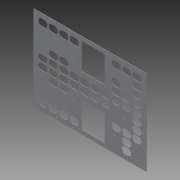
# Autodesk Inventor part: hybridbasearchive
Saved by Autodesk Inventor 2014 SP1 (Build 180222100, 222)
## iProperties
Created: 2014-01-05
Part Number: hybridbasearchive
Material: Aluminum 6061
Document SubType Name: Sheet Metal
Designer: Arpan
Density: 2.71 g/cm^3
Sheet Metal Rule: Default
Appearance: Aluminum - Flat
Mass: 1326.97 g
Surface Area: 6245.09 cm^2
Volume: 489.657 cm^3
Author: Arpan
Autodesk Inventor part; units mm, degrees
(part 1 of 2)
ref_plane "YZ Plane" through (0, 0, 0) normal (1, 0, 0) x (0, 1, 0)
ref_plane "XZ Plane" through (0, 0, 0) normal (0, 1, 0) x (-1, 0, 0)
ref_plane "XY Plane" through (0, 0, 0) normal (0, 0, 1) x (1, 0, 0)
sketch "Sketch1" plane through (0, 0, 0) normal (0, 0, 1) x (1, 0, 0)
  line L0 (0, 0) -> (-685.8, 0)
  line L1 (-685.8, 0) -> (-685.8, 516.255)
  line L2 (-685.8, 516.255) -> (0, 516.255)
  line L3 (0, 516.255) -> (0, 0)
  dimension "d0" = 685.8
  dimension "d1" = 516.255
  measures "d0" distance of L1.end L2.end
  measures "d1" distance of L2.end L0.start
extrude "Plate1" add sketch "Sketch1" along normal blind 1.5875
sketch "Sketch4" plane through (0, 0, 1.5875) normal (0, 0, 1) x (1, 0, 0)
  circle A0 centre (-673.1, 503.555) radius 2.0828 projected
  circle A1 centre (-673.1, 12.7) radius 2.0828 projected
extrude "Cut3" cut sketch "Sketch4" against normal blind 1.5875
pattern_linear "Rectangular Pattern2" count 27 spacing 25.4 along (1, 0, 0) of "Cut3"
sketch "Sketch2" plane through (0, 0, 1.5875) normal (0, 0, 1) x (1, 0, 0)
  line L0 (0, 0) -> (-685.8, 0) projected
  line L1 (-685.8, 516.255) -> (0, 516.255) projected
  line L2 (-342.9, 516.255) -> (-392.43, 516.255)
  line L3 (-392.43, 516.255) -> (-392.43, 332.105)
  line L4 (-392.43, 332.105) -> (-252.73, 332.105)
  line L5 (-252.73, 332.105) -> (-252.73, 516.255)
  line L6 (-392.43, 0) -> (-392.43, 184.15)
  line L7 (-392.43, 184.15) -> (-252.73, 184.15)
  line L8 (-252.73, 184.15) -> (-252.73, 0)
  line L9 (-392.43, 0) -> (-392.43, 25.4)
  line L10 (-392.43, 25.4) -> (-252.73, 25.4)
  line L11 (-252.73, 516.255) -> (-252.73, 490.855)
  line L12 (-252.73, 490.855) -> (-392.43, 490.855)
  line L13 (-685.8, 0) -> (-685.8, 516.255) projected
  dimension "d4" = 184.15
  dimension "d5" = 139.7
  dimension "d6" = 184.15
  dimension "d23" = 25.4
  dimension "d24" = 25.4
  dimension "d78" = 293.37
  dimension "d79" = 139.7
  dimension "d80" = 293.37
  constraints: 22 end point, 8 point on line, 6 perpendicular, 2 parallel, 1 midpoint
  measures "d4" distance of L2.end L3.end
  measures "d5" distance of L3.end L4.end
  measures "d6" distance of L6.start L6.end
  measures "d23" distance of L6.start L9.end
  measures "d24" distance of L5.end L11.end
  measures "d78" distance between parallel lines of L13 L6
  measures "d79" distance between parallel lines of L8 L6
  measures "d80" distance between parallel lines of L13 L3
extrude "Cut6" cut sketch "Sketch2" against normal blind 1.5875 contours L10 L6 L7 L8 | L12 L5 L4 L3
sketch "Sketch12" plane through (0, 0, 1.5875) normal (0, 0, 1) x (1, 0, 0)
  arc A0 (-673.1762, 31.5962) -> (-673.1762, 27.4588) centre (-673.1, 29.5275) ccw projected
  arc A1 (-673.0238, 27.4588) -> (-673.0238, 31.5962) centre (-673.1, 29.5275) ccw projected
  circle A2 centre (-673.1, 29.5275) radius 2.0701
  constraints: 1 centre point, 1 coincident, 1 concentric
extrude "Cut8" cut sketch "Sketch12" against normal blind 1.5875
pattern_linear "Rectangular Pattern5" count 19 spacing 25.4 along (0, 1, 0) count 2 spacing 660.4 along (1, 0, 0) of "Cut8"
sketch "Sketch16" plane through (0, 0, 1.5875) normal (0, 0, 1) x (1, 0, 0)
  line L0 (-685.8, 0) -> (-685.8, 516.255) projected
  line L1 (0, 516.255) -> (0, 0) projected
  circle A0 centre (-602.8344, 420.0249) radius 2.1723 projected
  circle A1 centre (-644.6428, 357.8965) radius 2.1989 projected
  circle A2 centre (-593.5881, 357.8965) radius 2.1989 projected
  circle A3 centre (-551.7797, 420.0249) radius 2.1723 projected
  circle A4 centre (-542.5208, 357.8965) radius 2.1989 projected
  circle A5 centre (-500.7124, 420.0249) radius 2.1723 projected
  circle A6 centre (-449.633, 420.0249) radius 2.1723 projected
  circle A7 centre (-491.4414, 357.8965) radius 2.1989 projected
  circle A8 centre (-440.3741, 357.8965) radius 2.1989 projected
  circle A9 centre (-398.5657, 420.0249) radius 2.1723 projected
  circle A10 centre (-417.8895, 321.6304) radius 3.2639 projected
  circle A11 centre (-417.8895, 194.6304) radius 3.2639 projected
  circle A12 centre (-627.4395, 321.6304) radius 3.2639 projected
  circle A13 centre (-627.4395, 194.6304) radius 3.2639 projected
  circle A14 centre (-644.6428, 96.019) radius 2.1989 projected
  circle A15 centre (-602.8344, 158.1474) radius 2.1723 projected
  circle A16 centre (-593.5881, 96.019) radius 2.1989 projected
  circle A17 centre (-551.7797, 158.1474) radius 2.1723 projected
  circle A18 centre (-542.5208, 96.019) radius 2.1989 projected
  circle A19 centre (-500.7124, 158.1474) radius 2.1723 projected
  circle A20 centre (-449.633, 158.1474) radius 2.1723 projected
  circle A21 centre (-491.4414, 96.019) radius 2.1989 projected
  circle A22 centre (-440.3741, 96.019) radius 2.1989 projected
  circle A23 centre (-398.5657, 158.1474) radius 2.1723 projected
  line L2 (-685.8, 258.1275) -> (0, 258.1275)
  circle A24 centre (-602.8344, 96.2301) radius 2.1723
  circle A25 centre (-644.6428, 158.3585) radius 2.1989
  circle A26 centre (-593.5881, 158.3585) radius 2.1989
  circle A27 centre (-551.7797, 96.2301) radius 2.1723
  circle A28 centre (-542.5208, 158.3585) radius 2.1989
  circle A29 centre (-500.7124, 96.2301) radius 2.1723
  circle A30 centre (-449.633, 96.2301) radius 2.1723
  circle A31 centre (-491.4414, 158.3585) radius 2.1989
  circle A32 centre (-440.3741, 158.3585) radius 2.1989
  circle A33 centre (-398.5657, 96.2301) radius 2.1723
  circle A34 centre (-644.6428, 420.236) radius 2.1989
  circle A35 centre (-602.8344, 358.1076) radius 2.1723
  circle A36 centre (-593.5881, 420.236) radius 2.1989
  circle A37 centre (-551.7797, 358.1076) radius 2.1723
  circle A38 centre (-542.5208, 420.236) radius 2.1989
  circle A39 centre (-500.7124, 358.1076) radius 2.1723
  circle A40 centre (-449.633, 358.1076) radius 2.1723
  circle A41 centre (-491.4414, 420.236) radius 2.1989
  circle A42 centre (-440.3741, 420.236) radius 2.1989
  circle A43 centre (-398.5657, 358.1076) radius 2.1723
  circle A44 centre (-133.294, 368.9594) radius 2.2479 projected
  circle A45 centre (-194.254, 368.9594) radius 1.5457 projected
  circle A46 centre (-196.794, 254.6594) radius 2.2655 projected
  circle A47 centre (-198.3647, 418.811) radius 2.5119 projected
  circle A48 centre (-151.1207, 418.811) radius 2.5119 projected
  circle A49 centre (-187.6385, 209.9079) radius 3.5177 projected
  circle A50 centre (-131.6773, 209.9079) radius 3.5177 projected
  circle A51 centre (-197.0948, 95.631) radius 2.4116 projected
  circle A52 centre (-197.0948, 59.563) radius 2.4116 projected
  circle A53 centre (-57.15, 57.15) radius 2.4116 projected
  circle A54 centre (-57.15, 98.044) radius 2.4116 projected
  constraints: 20 symmetric about line, 2 end point, 2 midpoint, 20 other
extrude "Cut9" cut sketch "Sketch16" against normal blind 1.5875 contours A0 | A1 | A2 | A3 | A4 | A5 | A6 | A7 | A8 | A9 | A10 | A11 | A12 | A13 | A14 | A15 | A16 | A17 | A18 | A19 | A20 | A21 | A22 | A23 | A24 | A25 | A26 | A27 | A28 | A29 | A30 | A31 | A32 | A33 | A34 | A35 | A36 | A37 | A38 | A39 | A40 | A41 | A42 | A43 | A44 | A46 | A47 | A48 | A49 | A50 | A51 | A52 | A53 | A54
sketch "Sketch17" plane through (0, 0, 1.5875) normal (0, 0, 1) x (1, 0, 0)
  line L0 (-685.8, 0) -> (-685.8, 516.255) projected
  line L1 (0, 0) -> (-685.8, 0) projected
  line L2 (0, 516.255) -> (0, 0) projected
  line L3 (-685.8, 516.255) -> (0, 516.255) projected
  line L4 (-685.8, 516.255) -> (0, 516.255)
  line L5 (0, 516.255) -> (0, 0)
  line L6 (0, 0) -> (-685.8, 0)
  line L7 (-685.8, 0) -> (-685.8, 516.255)
  line L8 (-25.4, 490.855) -> (-25.4, 25.4)
  line L9 (-25.4, 25.4) -> (-660.4, 25.4)
  line L10 (-660.4, 25.4) -> (-660.4, 490.855)
  line L11 (-660.4, 490.855) -> (-25.4, 490.855)
  circle A0 centre (-417.8895, 321.6304) radius 3.2639 projected
  circle A1 centre (-198.3647, 418.811) radius 2.5119 projected
  circle A2 centre (-440.3741, 420.236) radius 2.1989 projected
  circle A3 centre (-542.5208, 420.236) radius 2.1989 projected
  circle A4 centre (-644.6428, 420.236) radius 2.1989 projected
  circle A5 centre (-491.4414, 357.8965) radius 2.1989 projected
  circle A6 centre (-593.5881, 357.8965) radius 2.1989 projected
  circle A7 centre (-398.5657, 358.1076) radius 2.1723 projected
  circle A8 centre (-500.7124, 358.1076) radius 2.1723 projected
  circle A9 centre (-602.8344, 358.1076) radius 2.1723 projected
  circle A10 centre (-449.633, 420.0249) radius 2.1723 projected
  circle A11 centre (-551.7797, 420.0249) radius 2.1723 projected
  circle A12 centre (-131.6773, 209.9079) radius 3.5177 projected
  circle A13 centre (-627.4395, 194.6304) radius 3.2639 projected
  circle A14 centre (-57.15, 98.044) radius 2.4116 projected
  circle A15 centre (-197.0948, 59.563) radius 2.4116 projected
  circle A16 centre (-196.794, 254.6594) radius 2.2655 projected
  circle A17 centre (-542.5208, 158.3585) radius 2.1989 projected
  circle A18 centre (-491.4414, 158.3585) radius 2.1989 projected
  circle A19 centre (-440.3741, 96.019) radius 2.1989 projected
  circle A20 centre (-542.5208, 96.019) radius 2.1989 projected
  circle A21 centre (-644.6428, 96.019) radius 2.1989 projected
  circle A22 centre (-449.633, 96.2301) radius 2.1723 projected
  circle A23 centre (-500.7124, 96.2301) radius 2.1723 projected
  circle A24 centre (-398.5657, 158.1474) radius 2.1723 projected
  circle A25 centre (-500.7124, 158.1474) radius 2.1723 projected
  circle A26 centre (-602.8344, 158.1474) radius 2.1723 projected
  circle A27 centre (-551.7797, 158.1474) radius 2.1723 projected
  circle A28 centre (-449.633, 158.1474) radius 2.1723 projected
  circle A29 centre (-398.5657, 96.2301) radius 2.1723 projected
  circle A30 centre (-551.7797, 96.2301) radius 2.1723 projected
  circle A31 centre (-602.8344, 96.2301) radius 2.1723 projected
  circle A32 centre (-593.5881, 96.019) radius 2.1989 projected
  circle A33 centre (-491.4414, 96.019) radius 2.1989 projected
  circle A34 centre (-593.5881, 158.3585) radius 2.1989 projected
  circle A35 centre (-440.3741, 158.3585) radius 2.1989 projected
  circle A36 centre (-644.6428, 158.3585) radius 2.1989 projected
  circle A37 centre (-197.0948, 95.631) radius 2.4116 projected
  circle A38 centre (-57.15, 57.15) radius 2.4116 projected
  circle A39 centre (-417.8895, 194.6304) radius 3.2639 projected
  circle A40 centre (-187.6385, 209.9079) radius 3.5177 projected
  circle A41 centre (-602.8344, 420.0249) radius 2.1723 projected
  circle A42 centre (-500.7124, 420.0249) radius 2.1723 projected
  circle A43 centre (-398.5657, 420.0249) radius 2.1723 projected
  circle A44 centre (-551.7797, 358.1076) radius 2.1723 projected
  circle A45 centre (-449.633, 358.1076) radius 2.1723 projected
  circle A46 centre (-644.6428, 357.8965) radius 2.1989 projected
  circle A47 centre (-542.5208, 357.8965) radius 2.1989 projected
  circle A48 centre (-440.3741, 357.8965) radius 2.1989 projected
  circle A49 centre (-593.5881, 420.236) radius 2.1989 projected
  circle A50 centre (-491.4414, 420.236) radius 2.1989 projected
  circle A51 centre (-133.294, 368.9594) radius 2.2479 projected
  circle A52 centre (-151.1207, 418.811) radius 2.5119 projected
  circle A53 centre (-627.4395, 321.6304) radius 3.2639 projected
  circle A54 centre (-12.7, 486.7275) radius 2.0701 projected
  circle A55 centre (-12.7, 461.3275) radius 2.0701 projected
  circle A56 centre (-12.7, 435.9275) radius 2.0701 projected
  circle A57 centre (-12.7, 410.5275) radius 2.0701 projected
  circle A58 centre (-12.7, 385.1275) radius 2.0701 projected
  circle A59 centre (-12.7, 359.7275) radius 2.0701 projected
  circle A60 centre (-12.7, 334.3275) radius 2.0701 projected
  circle A61 centre (-12.7, 308.9275) radius 2.0701 projected
  circle A62 centre (-12.7, 283.5275) radius 2.0701 projected
  circle A63 centre (-12.7, 258.1275) radius 2.0701 projected
  circle A64 centre (-12.7, 232.7275) radius 2.0701 projected
  circle A65 centre (-12.7, 207.3275) radius 2.0701 projected
  circle A66 centre (-12.7, 181.9275) radius 2.0701 projected
  circle A67 centre (-12.7, 156.5275) radius 2.0701 projected
  circle A68 centre (-12.7, 131.1275) radius 2.0701 projected
  circle A69 centre (-12.7, 105.7275) radius 2.0701 projected
  circle A70 centre (-12.7, 80.3275) radius 2.0701 projected
  circle A71 centre (-12.7, 54.9275) radius 2.0701 projected
  circle A72 centre (-12.7, 29.5275) radius 2.0701 projected
  circle A73 centre (-673.1, 486.7275) radius 2.0701 projected
  circle A74 centre (-673.1, 461.3275) radius 2.0701 projected
  circle A75 centre (-673.1, 435.9275) radius 2.0701 projected
  circle A76 centre (-673.1, 410.5275) radius 2.0701 projected
  circle A77 centre (-673.1, 385.1275) radius 2.0701 projected
  circle A78 centre (-673.1, 359.7275) radius 2.0701 projected
  circle A79 centre (-673.1, 334.3275) radius 2.0701 projected
  circle A80 centre (-673.1, 308.9275) radius 2.0701 projected
  circle A81 centre (-673.1, 283.5275) radius 2.0701 projected
  circle A82 centre (-673.1, 258.1275) radius 2.0701 projected
  circle A83 centre (-673.1, 232.7275) radius 2.0701 projected
  circle A84 centre (-673.1, 207.3275) radius 2.0701 projected
  circle A85 centre (-673.1, 181.9275) radius 2.0701 projected
  circle A86 centre (-673.1, 156.5275) radius 2.0701 projected
  circle A87 centre (-673.1, 131.1275) radius 2.0701 projected
  circle A88 centre (-673.1, 105.7275) radius 2.0701 projected
  circle A89 centre (-673.1, 80.3275) radius 2.0701 projected
  circle A90 centre (-673.1, 54.9275) radius 2.0701 projected
  circle A91 centre (-673.1, 29.5275) radius 2.0701 projected
  line L12 (-252.73, 332.105) -> (-252.73, 490.855) projected
  line L13 (-252.73, 490.855) -> (-392.43, 490.855) projected
  line L14 (-392.43, 490.855) -> (-392.43, 332.105) projected
  line L15 (-392.43, 332.105) -> (-252.73, 332.105) projected
  line L16 (-392.43, 25.4) -> (-252.73, 25.4) projected
  line L17 (-252.73, 25.4) -> (-252.73, 184.15) projected
  line L18 (-252.73, 184.15) -> (-392.43, 184.15) projected
  line L19 (-392.43, 184.15) -> (-392.43, 25.4) projected
  circle A92 centre (-12.7, 503.555) radius 2.0828 projected
  circle A93 centre (-12.7, 12.7) radius 2.0828 projected
  circle A94 centre (-38.1, 503.555) radius 2.0828 projected
  circle A95 centre (-38.1, 12.7) radius 2.0828 projected
  circle A96 centre (-63.5, 503.555) radius 2.0828 projected
  circle A97 centre (-63.5, 12.7) radius 2.0828 projected
  circle A98 centre (-88.9, 503.555) radius 2.0828 projected
  circle A99 centre (-88.9, 12.7) radius 2.0828 projected
  circle A100 centre (-114.3, 503.555) radius 2.0828 projected
  circle A101 centre (-114.3, 12.7) radius 2.0828 projected
  circle A102 centre (-139.7, 503.555) radius 2.0828 projected
  circle A103 centre (-139.7, 12.7) radius 2.0828 projected
  circle A104 centre (-165.1, 503.555) radius 2.0828 projected
  circle A105 centre (-165.1, 12.7) radius 2.0828 projected
  circle A106 centre (-190.5, 503.555) radius 2.0828 projected
  circle A107 centre (-190.5, 12.7) radius 2.0828 projected
  circle A108 centre (-215.9, 503.555) radius 2.0828 projected
  circle A109 centre (-215.9, 12.7) radius 2.0828 projected
  circle A110 centre (-241.3, 503.555) radius 2.0828 projected
  circle A111 centre (-241.3, 12.7) radius 2.0828 projected
  circle A112 centre (-266.7, 503.555) radius 2.0828 projected
  circle A113 centre (-266.7, 12.7) radius 2.0828 projected
  circle A114 centre (-292.1, 503.555) radius 2.0828 projected
  circle A115 centre (-292.1, 12.7) radius 2.0828 projected
  circle A116 centre (-317.5, 503.555) radius 2.0828 projected
  circle A117 centre (-317.5, 12.7) radius 2.0828 projected
  circle A118 centre (-342.9, 503.555) radius 2.0828 projected
  circle A119 centre (-342.9, 12.7) radius 2.0828 projected
  circle A120 centre (-368.3, 503.555) radius 2.0828 projected
  circle A121 centre (-368.3, 12.7) radius 2.0828 projected
  circle A122 centre (-393.7, 503.555) radius 2.0828 projected
  circle A123 centre (-393.7, 12.7) radius 2.0828 projected
  circle A124 centre (-419.1, 503.555) radius 2.0828 projected
  circle A125 centre (-419.1, 12.7) radius 2.0828 projected
  circle A126 centre (-444.5, 503.555) radius 2.0828 projected
  circle A127 centre (-444.5, 12.7) radius 2.0828 projected
  circle A128 centre (-469.9, 503.555) radius 2.0828 projected
  circle A129 centre (-469.9, 12.7) radius 2.0828 projected
  circle A130 centre (-495.3, 503.555) radius 2.0828 projected
  circle A131 centre (-495.3, 12.7) radius 2.0828 projected
  circle A132 centre (-520.7, 503.555) radius 2.0828 projected
  circle A133 centre (-520.7, 12.7) radius 2.0828 projected
  circle A134 centre (-546.1, 503.555) radius 2.0828 projected
  circle A135 centre (-546.1, 12.7) radius 2.0828 projected
  circle A136 centre (-571.5, 503.555) radius 2.0828 projected
  circle A137 centre (-571.5, 12.7) radius 2.0828 projected
  circle A138 centre (-596.9, 503.555) radius 2.0828 projected
  circle A139 centre (-596.9, 12.7) radius 2.0828 projected
  circle A140 centre (-622.3, 503.555) radius 2.0828 projected
  circle A141 centre (-622.3, 12.7) radius 2.0828 projected
  circle A142 centre (-647.7, 503.555) radius 2.0828 projected
  circle A143 centre (-647.7, 12.7) radius 2.0828 projected
  circle A144 centre (-673.1, 503.555) radius 2.0828 projected
  circle A145 centre (-673.1, 12.7) radius 2.0828 projected
  line L20 (0, 0) -> (-685.8, 0) projected
  line L21 (-685.8, 0) -> (-685.8, 516.255) projected
  line L22 (-685.8, 516.255) -> (0, 516.255) projected
  line L23 (0, 516.255) -> (0, 0) projected
  line L24 (-108.6587, 162.306) -> (-32.6288, 162.306) projected
  line L25 (-111.4962, 162.306) -> (-115.8875, 162.306) projected
  arc A146 (-117.602, 164.0205) -> (-115.8875, 162.306) centre (-115.8875, 164.0205) ccw projected
  line L26 (-117.602, 164.0205) -> (-117.602, 350.7105) projected
  arc A147 (-115.8875, 352.425) -> (-117.602, 350.7105) centre (-115.8875, 350.7105) ccw projected
  line L27 (-115.8875, 352.425) -> (-111.4962, 352.425) projected
  line L28 (-111.4962, 352.425) -> (-108.6587, 352.425) projected
  line L29 (-32.6288, 352.425) -> (-108.6587, 352.425) projected
  line L30 (-129.655, 247.9766) -> (-200.4329, 247.9766) projected
  ellipse E0 centre (-200.4246, 251.0288) end of major axis (-202.5857, 248.8676) minor radius 3.048 (-203.4768, 251.0204) -> (-200.4329, 247.9766) ccw projected
  line L31 (-203.4768, 251.0204) -> (-203.4768, 372.5983) projected
  ellipse E1 centre (-200.4246, 372.59) end of major axis (-202.5857, 374.7512) minor radius 3.048 (-200.4329, 375.6422) -> (-203.4768, 372.5983) ccw projected
  line L32 (-200.4329, 375.6422) -> (-129.655, 375.6422) projected
  ellipse E2 centre (-129.6634, 372.59) end of major axis (-127.5022, 374.7512) minor radius 3.048 (-126.6112, 372.5983) -> (-129.655, 375.6422) ccw projected
  line L33 (-126.6112, 372.5983) -> (-126.6112, 251.0204) projected
  ellipse E3 centre (-129.6634, 251.0288) end of major axis (-127.5022, 248.8676) minor radius 3.048 (-129.655, 247.9766) -> (-126.6112, 251.0204) ccw projected
  line L34 (-129.655, 247.9766) -> (-200.4329, 247.9766) projected
  line L35 (-82.2426, 377.9851) -> (-122.6802, 377.9851) projected
  line L36 (-53.3399, 378.0501) -> (-79.1725, 378.0501)
  line L37 (-50.8, 462.8503) -> (-50.8, 380.5899) projected
  line L38 (-79.1725, 465.39) -> (-53.3399, 465.39) projected
  line L39 (-122.6802, 465.455) -> (-82.2426, 465.455) projected
  line L40 (-228.9463, 462.8619) -> (-228.9463, 380.5782) projected
  line L41 (-202.7682, 53.975) -> (-202.7682, 101.219) projected
  line L42 (-150.3807, 50.8) -> (-188.4807, 50.8) projected
  line L43 (-150.3807, 50.8) -> (-65.0875, 50.8)
  line L44 (-50.8, 101.219) -> (-50.8, 53.975) projected
  line L45 (-150.3807, 104.394) -> (-65.0875, 104.394)
  line L46 (-188.4807, 104.394) -> (-150.3807, 104.394) projected
  arc A148 (-199.5932, 104.394) -> (-202.7682, 101.219) centre (-199.5932, 101.219) ccw projected
  arc A149 (-202.7682, 53.975) -> (-199.5932, 50.8) centre (-199.5932, 53.975) ccw projected
  arc A150 (-53.975, 50.8) -> (-50.8, 53.975) centre (-53.975, 53.975) ccw projected
  arc A151 (-50.8, 101.219) -> (-53.975, 104.394) centre (-53.975, 101.219) ccw projected
  line L47 (-395.5303, 371.2862) -> (-395.5303, 406.6352) projected
  line L48 (-647.9194, 359.9754) -> (-647.9194, 419.9238) projected
  line L49 (-619.0742, 423.0821) -> (-644.3223, 423.0821) projected
  line L50 (-438.3523, 354.8393) -> (-398.8862, 354.8393) projected
  line L51 (-443.7909, 329.1941) -> (-619.3061, 329.1941) projected
  line L52 (-617.7043, 187.0668) -> (-442.0909, 187.0668) projected
  line L53 (-409.4461, 322.1471) -> (-409.4461, 194.1137) projected
  line L54 (-634.9475, 195.049) -> (-634.9475, 321.2118) projected
  line L55 (-395.5177, 109.4556) -> (-395.5177, 144.7108) projected
  line L56 (-647.6908, 144.7108) -> (-647.6908, 109.4556) projected
  line L57 (-619.0742, 161.2046) -> (-644.3223, 161.2046) projected
  line L58 (-438.3523, 92.9618) -> (-398.8862, 92.9618) projected
  line L59 (-660.4, 490.855) -> (-660.4, 444.3095)
  line L60 (-660.4, 444.3095) -> (-596.9, 444.3095)
  line L61 (-596.9, 444.3095) -> (-596.9, 490.855)
  line L62 (-660.4, 467.5822) -> (-596.9, 467.5822) construction
  line L63 (-637.1273, 444.3095) -> (-620.1728, 444.3095)
  line L64 (-620.1728, 490.855) -> (-637.1273, 490.855)
  arc A152 (-637.1273, 490.855) -> (-637.1273, 444.3095) centre (-637.1273, 467.5822) ccw
  arc A153 (-620.1728, 444.3095) -> (-620.1728, 490.855) centre (-620.1728, 467.5822) ccw
  line L65 (-620.1728, 487.68) -> (-637.1273, 487.68)
  arc A154 (-637.1273, 487.68) -> (-637.1273, 447.4845) centre (-637.1273, 467.5822) ccw
  line L66 (-637.1273, 447.4845) -> (-620.1728, 447.4845)
  arc A155 (-620.1728, 447.4845) -> (-620.1728, 487.68) centre (-620.1728, 467.5822) ccw
  line L67 (-620.1728, 441.1345) -> (-637.1273, 441.1345)
  arc A156 (-637.1273, 441.1345) -> (-637.1273, 400.939) centre (-637.1273, 421.0367) ccw
  line L68 (-637.1273, 400.939) -> (-620.1728, 400.939)
  arc A157 (-620.1728, 400.939) -> (-620.1728, 441.1345) centre (-620.1728, 421.0367) ccw
  line L69 (-620.1728, 394.589) -> (-637.1273, 394.589)
  arc A158 (-637.1273, 394.589) -> (-637.1273, 354.3935) centre (-637.1273, 374.4912) ccw
  line L70 (-637.1273, 354.3935) -> (-620.1728, 354.3935)
  arc A159 (-620.1728, 354.3935) -> (-620.1728, 394.589) centre (-620.1728, 374.4912) ccw
  line L71 (-620.1728, 348.0435) -> (-637.1273, 348.0435)
  arc A160 (-637.1273, 348.0435) -> (-637.1273, 307.848) centre (-637.1273, 327.9457) ccw
  line L72 (-637.1273, 307.848) -> (-620.1728, 307.848)
  arc A161 (-620.1728, 307.848) -> (-620.1728, 348.0435) centre (-620.1727, 327.9457) ccw
  line L73 (-620.1728, 301.498) -> (-637.1273, 301.498)
  arc A162 (-637.1273, 301.498) -> (-637.1273, 261.3025) centre (-637.1273, 281.4002) ccw
  line L74 (-637.1273, 261.3025) -> (-620.1728, 261.3025)
  arc A163 (-620.1728, 261.3025) -> (-620.1728, 301.498) centre (-620.1727, 281.4002) ccw
  line L75 (-620.1728, 254.9525) -> (-637.1273, 254.9525)
  arc A164 (-637.1273, 254.9525) -> (-637.1273, 214.757) centre (-637.1273, 234.8547) ccw
  line L76 (-637.1273, 214.757) -> (-620.1728, 214.757)
  arc A165 (-620.1728, 214.757) -> (-620.1728, 254.9525) centre (-620.1727, 234.8547) ccw
  line L77 (-620.1728, 208.407) -> (-637.1273, 208.407)
  arc A166 (-637.1273, 208.407) -> (-637.1273, 168.2115) centre (-637.1273, 188.3092) ccw
  line L78 (-637.1273, 168.2115) -> (-620.1728, 168.2115)
  arc A167 (-620.1728, 168.2115) -> (-620.1728, 208.407) centre (-620.1727, 188.3092) ccw
  line L79 (-620.1728, 161.8615) -> (-637.1273, 161.8615)
  arc A168 (-637.1273, 161.8615) -> (-637.1273, 121.666) centre (-637.1273, 141.7637) ccw
  line L80 (-637.1273, 121.666) -> (-620.1728, 121.666)
  arc A169 (-620.1728, 121.666) -> (-620.1728, 161.8615) centre (-620.1727, 141.7637) ccw
  line L81 (-620.1728, 115.316) -> (-637.1273, 115.316)
  arc A170 (-637.1273, 115.316) -> (-637.1273, 75.1205) centre (-637.1273, 95.2182) ccw
  line L82 (-637.1273, 75.1205) -> (-620.1728, 75.1205)
  arc A171 (-620.1728, 75.1205) -> (-620.1728, 115.316) centre (-620.1727, 95.2182) ccw
  line L83 (-620.1728, 68.7705) -> (-637.1272, 68.7705)
  arc A172 (-637.1272, 68.7705) -> (-637.1272, 28.575) centre (-637.1272, 48.6727) ccw
  line L84 (-637.1272, 28.575) -> (-620.1728, 28.575)
  arc A173 (-620.1728, 28.575) -> (-620.1728, 68.7705) centre (-620.1727, 48.6727) ccw
  line L85 (-556.6728, 487.68) -> (-573.6273, 487.68)
  arc A174 (-573.6273, 487.68) -> (-573.6273, 447.4845) centre (-573.6273, 467.5822) ccw
  line L86 (-573.6273, 447.4845) -> (-556.6728, 447.4845)
  arc A175 (-556.6728, 447.4845) -> (-556.6728, 487.68) centre (-556.6728, 467.5822) ccw
  line L87 (-556.6728, 441.1345) -> (-573.6273, 441.1345)
  arc A176 (-573.6273, 441.1345) -> (-573.6273, 400.939) centre (-573.6273, 421.0367) ccw
  line L88 (-573.6273, 400.939) -> (-556.6728, 400.939)
  arc A177 (-556.6728, 400.939) -> (-556.6728, 441.1345) centre (-556.6728, 421.0367) ccw
  line L89 (-556.6728, 394.589) -> (-573.6273, 394.589)
  arc A178 (-573.6273, 394.589) -> (-573.6273, 354.3935) centre (-573.6273, 374.4912) ccw
  line L90 (-573.6273, 354.3935) -> (-556.6728, 354.3935)
  arc A179 (-556.6728, 354.3935) -> (-556.6728, 394.589) centre (-556.6728, 374.4912) ccw
  line L91 (-556.6728, 348.0435) -> (-573.6273, 348.0435)
  arc A180 (-573.6273, 348.0435) -> (-573.6273, 307.848) centre (-573.6273, 327.9457) ccw
  line L92 (-573.6273, 307.848) -> (-556.6728, 307.848)
  arc A181 (-556.6728, 307.848) -> (-556.6728, 348.0435) centre (-556.6728, 327.9457) ccw
  line L93 (-556.6728, 301.498) -> (-573.6273, 301.498)
  arc A182 (-573.6273, 301.498) -> (-573.6273, 261.3025) centre (-573.6273, 281.4002) ccw
  line L94 (-573.6273, 261.3025) -> (-556.6728, 261.3025)
  arc A183 (-556.6728, 261.3025) -> (-556.6728, 301.498) centre (-556.6728, 281.4002) ccw
  line L95 (-556.6728, 254.9525) -> (-573.6273, 254.9525)
  arc A184 (-573.6273, 254.9525) -> (-573.6273, 214.757) centre (-573.6273, 234.8547) ccw
  line L96 (-573.6273, 214.757) -> (-556.6728, 214.757)
  arc A185 (-556.6728, 214.757) -> (-556.6728, 254.9525) centre (-556.6727, 234.8547) ccw
  line L97 (-556.6728, 208.407) -> (-573.6273, 208.407)
  arc A186 (-573.6273, 208.407) -> (-573.6273, 168.2115) centre (-573.6273, 188.3092) ccw
  line L98 (-573.6273, 168.2115) -> (-556.6728, 168.2115)
  arc A187 (-556.6728, 168.2115) -> (-556.6728, 208.407) centre (-556.6727, 188.3092) ccw
  line L99 (-556.6728, 161.8615) -> (-573.6273, 161.8615)
  arc A188 (-573.6273, 161.8615) -> (-573.6273, 121.666) centre (-573.6273, 141.7637) ccw
  line L100 (-573.6273, 121.666) -> (-556.6728, 121.666)
  arc A189 (-556.6728, 121.666) -> (-556.6728, 161.8615) centre (-556.6727, 141.7637) ccw
  line L101 (-556.6728, 115.316) -> (-573.6273, 115.316)
  arc A190 (-573.6273, 115.316) -> (-573.6273, 75.1205) centre (-573.6273, 95.2182) ccw
  line L102 (-573.6273, 75.1205) -> (-556.6728, 75.1205)
  arc A191 (-556.6728, 75.1205) -> (-556.6728, 115.316) centre (-556.6727, 95.2182) ccw
  line L103 (-556.6728, 68.7705) -> (-573.6273, 68.7705)
  arc A192 (-573.6273, 68.7705) -> (-573.6273, 28.575) centre (-573.6273, 48.6727) ccw
  line L104 (-573.6273, 28.575) -> (-556.6728, 28.575)
  arc A193 (-556.6728, 28.575) -> (-556.6728, 68.7705) centre (-556.6727, 48.6727) ccw
  line L105 (-493.1728, 487.68) -> (-510.1273, 487.68)
  arc A194 (-510.1273, 487.68) -> (-510.1273, 447.4845) centre (-510.1273, 467.5822) ccw
  line L106 (-510.1273, 447.4845) -> (-493.1728, 447.4845)
  arc A195 (-493.1728, 447.4845) -> (-493.1728, 487.68) centre (-493.1728, 467.5822) ccw
  line L107 (-493.1728, 441.1345) -> (-510.1273, 441.1345)
  arc A196 (-510.1273, 441.1345) -> (-510.1273, 400.939) centre (-510.1273, 421.0367) ccw
  line L108 (-510.1273, 400.939) -> (-493.1728, 400.939)
  arc A197 (-493.1728, 400.939) -> (-493.1728, 441.1345) centre (-493.1728, 421.0367) ccw
  line L109 (-493.1728, 394.589) -> (-510.1273, 394.589)
  arc A198 (-510.1273, 394.589) -> (-510.1273, 354.3935) centre (-510.1273, 374.4912) ccw
  line L110 (-510.1273, 354.3935) -> (-493.1728, 354.3935)
  arc A199 (-493.1728, 354.3935) -> (-493.1728, 394.589) centre (-493.1728, 374.4912) ccw
  line L111 (-493.1728, 348.0435) -> (-510.1273, 348.0435)
  arc A200 (-510.1273, 348.0435) -> (-510.1273, 307.848) centre (-510.1273, 327.9457) ccw
  line L112 (-510.1273, 307.848) -> (-493.1728, 307.848)
  arc A201 (-493.1728, 307.848) -> (-493.1728, 348.0435) centre (-493.1728, 327.9457) ccw
  line L113 (-493.1728, 301.498) -> (-510.1273, 301.498)
  arc A202 (-510.1273, 301.498) -> (-510.1273, 261.3025) centre (-510.1273, 281.4002) ccw
  line L114 (-510.1273, 261.3025) -> (-493.1728, 261.3025)
  arc A203 (-493.1728, 261.3025) -> (-493.1728, 301.498) centre (-493.1728, 281.4002) ccw
  line L115 (-493.1728, 254.9525) -> (-510.1273, 254.9525)
  arc A204 (-510.1273, 254.9525) -> (-510.1273, 214.757) centre (-510.1273, 234.8547) ccw
  line L116 (-510.1273, 214.757) -> (-493.1728, 214.757)
  arc A205 (-493.1728, 214.757) -> (-493.1728, 254.9525) centre (-493.1727, 234.8547) ccw
  line L117 (-493.1728, 208.407) -> (-510.1273, 208.407)
  arc A206 (-510.1273, 208.407) -> (-510.1273, 168.2115) centre (-510.1273, 188.3092) ccw
  line L118 (-510.1273, 168.2115) -> (-493.1728, 168.2115)
  arc A207 (-493.1728, 168.2115) -> (-493.1728, 208.407) centre (-493.1727, 188.3092) ccw
  line L119 (-493.1728, 161.8615) -> (-510.1272, 161.8615)
  arc A208 (-510.1272, 161.8615) -> (-510.1272, 121.666) centre (-510.1272, 141.7637) ccw
  line L120 (-510.1272, 121.666) -> (-493.1728, 121.666)
  arc A209 (-493.1728, 121.666) -> (-493.1728, 161.8615) centre (-493.1727, 141.7637) ccw
  line L121 (-493.1728, 115.316) -> (-510.1272, 115.316)
  arc A210 (-510.1272, 115.316) -> (-510.1272, 75.1205) centre (-510.1272, 95.2182) ccw
  line L122 (-510.1272, 75.1205) -> (-493.1728, 75.1205)
  arc A211 (-493.1728, 75.1205) -> (-493.1728, 115.316) centre (-493.1727, 95.2182) ccw
  line L123 (-493.1728, 68.7705) -> (-510.1272, 68.7705)
  arc A212 (-510.1272, 68.7705) -> (-510.1272, 28.575) centre (-510.1272, 48.6727) ccw
  line L124 (-510.1272, 28.575) -> (-493.1728, 28.575)
  arc A213 (-493.1728, 28.575) -> (-493.1728, 68.7705) centre (-493.1727, 48.6727) ccw
  line L125 (-429.6728, 487.68) -> (-446.6273, 487.68)
  arc A214 (-446.6273, 487.68) -> (-446.6273, 447.4845) centre (-446.6273, 467.5822) ccw
  line L126 (-446.6273, 447.4845) -> (-429.6728, 447.4845)
  arc A215 (-429.6728, 447.4845) -> (-429.6728, 487.68) centre (-429.6728, 467.5822) ccw
  line L127 (-429.6728, 441.1345) -> (-446.6273, 441.1345)
  arc A216 (-446.6273, 441.1345) -> (-446.6273, 400.939) centre (-446.6273, 421.0367) ccw
  line L128 (-446.6273, 400.939) -> (-429.6728, 400.939)
  arc A217 (-429.6728, 400.939) -> (-429.6728, 441.1345) centre (-429.6728, 421.0367) ccw
  line L129 (-429.6728, 394.589) -> (-446.6273, 394.589)
  arc A218 (-446.6273, 394.589) -> (-446.6273, 354.3935) centre (-446.6273, 374.4912) ccw
  line L130 (-446.6273, 354.3935) -> (-429.6728, 354.3935)
  arc A219 (-429.6728, 354.3935) -> (-429.6728, 394.589) centre (-429.6728, 374.4912) ccw
  line L131 (-429.6728, 348.0435) -> (-446.6273, 348.0435)
  arc A220 (-446.6273, 348.0435) -> (-446.6273, 307.848) centre (-446.6273, 327.9457) ccw
  line L132 (-446.6273, 307.848) -> (-429.6728, 307.848)
  arc A221 (-429.6728, 307.848) -> (-429.6728, 348.0435) centre (-429.6728, 327.9457) ccw
  line L133 (-429.6728, 301.498) -> (-446.6273, 301.498)
  arc A222 (-446.6273, 301.498) -> (-446.6273, 261.3025) centre (-446.6273, 281.4002) ccw
  line L134 (-446.6273, 261.3025) -> (-429.6728, 261.3025)
  arc A223 (-429.6728, 261.3025) -> (-429.6728, 301.498) centre (-429.6728, 281.4002) ccw
  line L135 (-429.6728, 254.9525) -> (-446.6273, 254.9525)
  arc A224 (-446.6273, 254.9525) -> (-446.6273, 214.757) centre (-446.6273, 234.8547) ccw
  line L136 (-446.6273, 214.757) -> (-429.6728, 214.757)
  arc A225 (-429.6728, 214.757) -> (-429.6728, 254.9525) centre (-429.6728, 234.8547) ccw
  line L137 (-429.6728, 208.407) -> (-446.6273, 208.407)
  arc A226 (-446.6273, 208.407) -> (-446.6273, 168.2115) centre (-446.6273, 188.3092) ccw
  line L138 (-446.6273, 168.2115) -> (-429.6728, 168.2115)
  arc A227 (-429.6728, 168.2115) -> (-429.6728, 208.407) centre (-429.6728, 188.3092) ccw
  line L139 (-429.6728, 161.8615) -> (-446.6272, 161.8615)
  arc A228 (-446.6272, 161.8615) -> (-446.6272, 121.666) centre (-446.6272, 141.7637) ccw
  line L140 (-446.6272, 121.666) -> (-429.6728, 121.666)
  arc A229 (-429.6728, 121.666) -> (-429.6728, 161.8615) centre (-429.6728, 141.7637) ccw
  line L141 (-429.6728, 115.316) -> (-446.6272, 115.316)
  arc A230 (-446.6272, 115.316) -> (-446.6272, 75.1205) centre (-446.6272, 95.2182) ccw
  line L142 (-446.6272, 75.1205) -> (-429.6728, 75.1205)
  arc A231 (-429.6728, 75.1205) -> (-429.6728, 115.316) centre (-429.6728, 95.2182) ccw
  line L143 (-429.6728, 68.7705) -> (-446.6272, 68.7705)
  arc A232 (-446.6272, 68.7705) -> (-446.6272, 28.575) centre (-446.6272, 48.6727) ccw
  line L144 (-446.6272, 28.575) -> (-429.6728, 28.575)
  arc A233 (-429.6728, 28.575) -> (-429.6728, 68.7705) centre (-429.6728, 48.6727) ccw
  line L145 (-366.1728, 487.68) -> (-383.1273, 487.68)
  arc A234 (-383.1273, 487.68) -> (-383.1273, 447.4845) centre (-383.1273, 467.5822) ccw
  line L146 (-383.1273, 447.4845) -> (-366.1728, 447.4845)
  arc A235 (-366.1728, 447.4845) -> (-366.1728, 487.68) centre (-366.1728, 467.5822) ccw
  line L147 (-366.1728, 441.1345) -> (-383.1273, 441.1345)
  arc A236 (-383.1273, 441.1345) -> (-383.1273, 400.939) centre (-383.1273, 421.0367) ccw
  line L148 (-383.1273, 400.939) -> (-366.1728, 400.939)
  arc A237 (-366.1728, 400.939) -> (-366.1728, 441.1345) centre (-366.1728, 421.0367) ccw
  line L149 (-366.1728, 394.589) -> (-383.1273, 394.589)
  arc A238 (-383.1273, 394.589) -> (-383.1273, 354.3935) centre (-383.1273, 374.4912) ccw
  line L150 (-383.1273, 354.3935) -> (-366.1728, 354.3935)
  arc A239 (-366.1728, 354.3935) -> (-366.1728, 394.589) centre (-366.1728, 374.4912) ccw
  line L151 (-366.1728, 348.0435) -> (-383.1273, 348.0435)
  arc A240 (-383.1273, 348.0435) -> (-383.1273, 307.848) centre (-383.1273, 327.9457) ccw
  line L152 (-383.1273, 307.848) -> (-366.1728, 307.848)
  arc A241 (-366.1728, 307.848) -> (-366.1728, 348.0435) centre (-366.1728, 327.9457) ccw
  line L153 (-366.1728, 301.498) -> (-383.1273, 301.498)
  arc A242 (-383.1273, 301.498) -> (-383.1273, 261.3025) centre (-383.1273, 281.4002) ccw
  line L154 (-383.1273, 261.3025) -> (-366.1728, 261.3025)
  arc A243 (-366.1728, 261.3025) -> (-366.1728, 301.498) centre (-366.1728, 281.4002) ccw
  line L155 (-366.1728, 254.9525) -> (-383.1273, 254.9525)
  arc A244 (-383.1273, 254.9525) -> (-383.1273, 214.757) centre (-383.1273, 234.8547) ccw
  line L156 (-383.1273, 214.757) -> (-366.1728, 214.757)
  arc A245 (-366.1728, 214.757) -> (-366.1728, 254.9525) centre (-366.1728, 234.8547) ccw
  line L157 (-366.1728, 208.407) -> (-383.1273, 208.407)
  arc A246 (-383.1273, 208.407) -> (-383.1273, 168.2115) centre (-383.1273, 188.3092) ccw
  line L158 (-383.1273, 168.2115) -> (-366.1728, 168.2115)
  arc A247 (-366.1728, 168.2115) -> (-366.1728, 208.407) centre (-366.1728, 188.3092) ccw
  line L159 (-366.1728, 161.8615) -> (-383.1273, 161.8615)
  arc A248 (-383.1273, 161.8615) -> (-383.1273, 121.666) centre (-383.1273, 141.7637) ccw
  line L160 (-383.1273, 121.666) -> (-366.1728, 121.666)
  arc A249 (-366.1728, 121.666) -> (-366.1728, 161.8615) centre (-366.1727, 141.7637) ccw
  line L161 (-366.1728, 115.316) -> (-383.1273, 115.316)
  arc A250 (-383.1273, 115.316) -> (-383.1273, 75.1205) centre (-383.1273, 95.2182) ccw
  line L162 (-383.1273, 75.1205) -> (-366.1728, 75.1205)
  arc A251 (-366.1728, 75.1205) -> (-366.1728, 115.316) centre (-366.1727, 95.2182) ccw
  line L163 (-366.1728, 68.7705) -> (-383.1273, 68.7705)
  arc A252 (-383.1273, 68.7705) -> (-383.1273, 28.575) centre (-383.1273, 48.6727) ccw
  line L164 (-383.1273, 28.575) -> (-366.1728, 28.575)
  arc A253 (-366.1728, 28.575) -> (-366.1728, 68.7705) centre (-366.1727, 48.6727) ccw
  line L165 (-302.6728, 487.68) -> (-319.6273, 487.68)
  arc A254 (-319.6273, 487.68) -> (-319.6273, 447.4845) centre (-319.6273, 467.5822) ccw
  line L166 (-319.6273, 447.4845) -> (-302.6728, 447.4845)
  arc A255 (-302.6728, 447.4845) -> (-302.6728, 487.68) centre (-302.6728, 467.5822) ccw
  line L167 (-302.6728, 441.1345) -> (-319.6273, 441.1345)
  arc A256 (-319.6273, 441.1345) -> (-319.6273, 400.939) centre (-319.6273, 421.0367) ccw
  line L168 (-319.6273, 400.939) -> (-302.6728, 400.939)
  arc A257 (-302.6728, 400.939) -> (-302.6728, 441.1345) centre (-302.6728, 421.0367) ccw
  line L169 (-302.6728, 394.589) -> (-319.6273, 394.589)
  arc A258 (-319.6273, 394.589) -> (-319.6273, 354.3935) centre (-319.6273, 374.4912) ccw
  line L170 (-319.6273, 354.3935) -> (-302.6728, 354.3935)
  arc A259 (-302.6728, 354.3935) -> (-302.6728, 394.589) centre (-302.6728, 374.4912) ccw
  line L171 (-302.6728, 348.0435) -> (-319.6273, 348.0435)
  arc A260 (-319.6273, 348.0435) -> (-319.6273, 307.848) centre (-319.6273, 327.9457) ccw
  line L172 (-319.6273, 307.848) -> (-302.6728, 307.848)
  arc A261 (-302.6728, 307.848) -> (-302.6728, 348.0435) centre (-302.6728, 327.9457) ccw
  line L173 (-302.6728, 301.498) -> (-319.6273, 301.498)
  arc A262 (-319.6273, 301.498) -> (-319.6273, 261.3025) centre (-319.6273, 281.4002) ccw
  line L174 (-319.6273, 261.3025) -> (-302.6728, 261.3025)
  arc A263 (-302.6728, 261.3025) -> (-302.6728, 301.498) centre (-302.6728, 281.4002) ccw
  line L175 (-302.6728, 254.9525) -> (-319.6273, 254.9525)
  arc A264 (-319.6273, 254.9525) -> (-319.6273, 214.757) centre (-319.6273, 234.8547) ccw
  line L176 (-319.6273, 214.757) -> (-302.6728, 214.757)
  arc A265 (-302.6728, 214.757) -> (-302.6728, 254.9525) centre (-302.6727, 234.8547) ccw
  line L177 (-302.6728, 208.407) -> (-319.6273, 208.407)
  arc A266 (-319.6273, 208.407) -> (-319.6273, 168.2115) centre (-319.6273, 188.3092) ccw
  line L178 (-319.6273, 168.2115) -> (-302.6728, 168.2115)
  arc A267 (-302.6728, 168.2115) -> (-302.6728, 208.407) centre (-302.6727, 188.3092) ccw
  line L179 (-302.6728, 161.8615) -> (-319.6272, 161.8615)
  arc A268 (-319.6272, 161.8615) -> (-319.6272, 121.666) centre (-319.6272, 141.7637) ccw
  line L180 (-319.6272, 121.666) -> (-302.6728, 121.666)
  arc A269 (-302.6728, 121.666) -> (-302.6728, 161.8615) centre (-302.6727, 141.7637) ccw
  line L181 (-302.6728, 115.316) -> (-319.6272, 115.316)
  arc A270 (-319.6272, 115.316) -> (-319.6272, 75.1205) centre (-319.6272, 95.2182) ccw
  line L182 (-319.6272, 75.1205) -> (-302.6728, 75.1205)
  arc A271 (-302.6728, 75.1205) -> (-302.6728, 115.316) centre (-302.6727, 95.2182) ccw
  line L183 (-302.6728, 68.7705) -> (-319.6272, 68.7705)
  arc A272 (-319.6272, 68.7705) -> (-319.6272, 28.575) centre (-319.6272, 48.6727) ccw
  line L184 (-319.6272, 28.575) -> (-302.6728, 28.575)
  arc A273 (-302.6728, 28.575) -> (-302.6728, 68.7705) centre (-302.6727, 48.6727) ccw
  line L185 (-239.1728, 487.68) -> (-256.1273, 487.68)
  arc A274 (-256.1273, 487.68) -> (-256.1273, 447.4845) centre (-256.1273, 467.5822) ccw
  line L186 (-256.1273, 447.4845) -> (-239.1728, 447.4845)
  arc A275 (-239.1728, 447.4845) -> (-239.1728, 487.68) centre (-239.1728, 467.5822) ccw
  line L187 (-239.1728, 441.1345) -> (-256.1273, 441.1345)
  arc A276 (-256.1273, 441.1345) -> (-256.1273, 400.939) centre (-256.1273, 421.0367) ccw
  line L188 (-256.1273, 400.939) -> (-239.1728, 400.939)
  arc A277 (-239.1728, 400.939) -> (-239.1728, 441.1345) centre (-239.1728, 421.0367) ccw
  line L189 (-239.1728, 394.589) -> (-256.1273, 394.589)
  arc A278 (-256.1273, 394.589) -> (-256.1273, 354.3935) centre (-256.1273, 374.4912) ccw
  line L190 (-256.1273, 354.3935) -> (-239.1728, 354.3935)
  arc A279 (-239.1728, 354.3935) -> (-239.1728, 394.589) centre (-239.1728, 374.4912) ccw
  line L191 (-239.1728, 348.0435) -> (-256.1273, 348.0435)
  arc A280 (-256.1273, 348.0435) -> (-256.1273, 307.848) centre (-256.1273, 327.9457) ccw
  line L192 (-256.1273, 307.848) -> (-239.1728, 307.848)
  arc A281 (-239.1728, 307.848) -> (-239.1728, 348.0435) centre (-239.1728, 327.9457) ccw
  line L193 (-239.1728, 301.498) -> (-256.1273, 301.498)
  arc A282 (-256.1273, 301.498) -> (-256.1273, 261.3025) centre (-256.1273, 281.4002) ccw
  line L194 (-256.1273, 261.3025) -> (-239.1728, 261.3025)
  arc A283 (-239.1728, 261.3025) -> (-239.1728, 301.498) centre (-239.1728, 281.4002) ccw
  line L195 (-239.1728, 254.9525) -> (-256.1273, 254.9525)
  arc A284 (-256.1273, 254.9525) -> (-256.1273, 214.757) centre (-256.1273, 234.8547) ccw
  line L196 (-256.1273, 214.757) -> (-239.1728, 214.757)
  arc A285 (-239.1728, 214.757) -> (-239.1728, 254.9525) centre (-239.1728, 234.8547) ccw
  line L197 (-239.1728, 208.407) -> (-256.1273, 208.407)
  arc A286 (-256.1273, 208.407) -> (-256.1273, 168.2115) centre (-256.1273, 188.3092) ccw
  line L198 (-256.1273, 168.2115) -> (-239.1728, 168.2115)
  arc A287 (-239.1728, 168.2115) -> (-239.1728, 208.407) centre (-239.1728, 188.3092) ccw
  line L199 (-239.1728, 161.8615) -> (-256.1273, 161.8615)
  arc A288 (-256.1273, 161.8615) -> (-256.1273, 121.666) centre (-256.1273, 141.7637) ccw
  line L200 (-256.1273, 121.666) -> (-239.1728, 121.666)
  arc A289 (-239.1728, 121.666) -> (-239.1728, 161.8615) centre (-239.1728, 141.7637) ccw
  line L201 (-239.1728, 115.316) -> (-256.1273, 115.316)
  arc A290 (-256.1273, 115.316) -> (-256.1273, 75.1205) centre (-256.1273, 95.2182) ccw
  line L202 (-256.1273, 75.1205) -> (-239.1728, 75.1205)
  arc A291 (-239.1728, 75.1205) -> (-239.1728, 115.316) centre (-239.1728, 95.2182) ccw
  line L203 (-239.1728, 68.7705) -> (-256.1273, 68.7705)
  arc A292 (-256.1273, 68.7705) -> (-256.1273, 28.575) centre (-256.1273, 48.6727) ccw
  line L204 (-256.1273, 28.575) -> (-239.1728, 28.575)
  arc A293 (-239.1728, 28.575) -> (-239.1728, 68.7705) centre (-239.1727, 48.6727) ccw
  line L205 (-175.6728, 487.68) -> (-192.6273, 487.68)
  arc A294 (-192.6273, 487.68) -> (-192.6273, 447.4845) centre (-192.6273, 467.5822) ccw
  line L206 (-192.6273, 447.4845) -> (-175.6728, 447.4845)
  arc A295 (-175.6728, 447.4845) -> (-175.6728, 487.68) centre (-175.6728, 467.5822) ccw
  line L207 (-175.6728, 441.1345) -> (-192.6273, 441.1345)
  arc A296 (-192.6273, 441.1345) -> (-192.6273, 400.939) centre (-192.6273, 421.0367) ccw
  line L208 (-192.6273, 400.939) -> (-175.6728, 400.939)
  arc A297 (-175.6728, 400.939) -> (-175.6728, 441.1345) centre (-175.6728, 421.0367) ccw
  line L209 (-175.6728, 394.589) -> (-192.6273, 394.589)
  arc A298 (-192.6273, 394.589) -> (-192.6273, 354.3935) centre (-192.6273, 374.4912) ccw
  line L210 (-192.6273, 354.3935) -> (-175.6728, 354.3935)
  arc A299 (-175.6728, 354.3935) -> (-175.6728, 394.589) centre (-175.6728, 374.4912) ccw
  line L211 (-175.6728, 348.0435) -> (-192.6273, 348.0435)
  arc A300 (-192.6273, 348.0435) -> (-192.6273, 307.848) centre (-192.6273, 327.9457) ccw
  line L212 (-192.6273, 307.848) -> (-175.6728, 307.848)
  arc A301 (-175.6728, 307.848) -> (-175.6728, 348.0435) centre (-175.6728, 327.9457) ccw
  line L213 (-175.6728, 301.498) -> (-192.6273, 301.498)
  arc A302 (-192.6273, 301.498) -> (-192.6273, 261.3025) centre (-192.6273, 281.4002) ccw
  line L214 (-192.6273, 261.3025) -> (-175.6728, 261.3025)
  arc A303 (-175.6728, 261.3025) -> (-175.6728, 301.498) centre (-175.6728, 281.4002) ccw
  line L215 (-175.6728, 254.9525) -> (-192.6273, 254.9525)
  arc A304 (-192.6273, 254.9525) -> (-192.6273, 214.757) centre (-192.6273, 234.8547) ccw
  line L216 (-192.6273, 214.757) -> (-175.6728, 214.757)
  arc A305 (-175.6728, 214.757) -> (-175.6728, 254.9525) centre (-175.6728, 234.8547) ccw
  line L217 (-175.6728, 208.407) -> (-192.6273, 208.407)
  arc A306 (-192.6273, 208.407) -> (-192.6273, 168.2115) centre (-192.6273, 188.3092) ccw
  line L218 (-192.6273, 168.2115) -> (-175.6728, 168.2115)
  arc A307 (-175.6728, 168.2115) -> (-175.6728, 208.407) centre (-175.6728, 188.3092) ccw
  line L219 (-175.6728, 161.8615) -> (-192.6273, 161.8615)
  arc A308 (-192.6273, 161.8615) -> (-192.6273, 121.666) centre (-192.6273, 141.7637) ccw
  line L220 (-192.6273, 121.666) -> (-175.6728, 121.666)
  arc A309 (-175.6728, 121.666) -> (-175.6728, 161.8615) centre (-175.6728, 141.7637) ccw
  line L221 (-175.6728, 115.316) -> (-192.6273, 115.316)
  arc A310 (-192.6273, 115.316) -> (-192.6273, 75.1205) centre (-192.6273, 95.2182) ccw
  line L222 (-192.6273, 75.1205) -> (-175.6728, 75.1205)
  arc A311 (-175.6728, 75.1205) -> (-175.6728, 115.316) centre (-175.6728, 95.2182) ccw
  line L223 (-175.6728, 68.7705) -> (-192.6272, 68.7705)
  arc A312 (-192.6272, 68.7705) -> (-192.6272, 28.575) centre (-192.6272, 48.6727) ccw
  line L224 (-192.6272, 28.575) -> (-175.6728, 28.575)
  arc A313 (-175.6728, 28.575) -> (-175.6728, 68.7705) centre (-175.6727, 48.6727) ccw
  line L225 (-112.1728, 487.68) -> (-129.1273, 487.68)
  arc A314 (-129.1273, 487.68) -> (-129.1273, 447.4845) centre (-129.1273, 467.5822) ccw
  line L226 (-129.1273, 447.4845) -> (-112.1728, 447.4845)
  arc A315 (-112.1728, 447.4845) -> (-112.1728, 487.68) centre (-112.1728, 467.5822) ccw
  line L227 (-112.1728, 441.1345) -> (-129.1273, 441.1345)
  arc A316 (-129.1273, 441.1345) -> (-129.1273, 400.939) centre (-129.1273, 421.0367) ccw
  line L228 (-129.1273, 400.939) -> (-112.1728, 400.939)
  arc A317 (-112.1728, 400.939) -> (-112.1728, 441.1345) centre (-112.1728, 421.0367) ccw
  line L229 (-112.1728, 394.589) -> (-129.1273, 394.589)
  arc A318 (-129.1273, 394.589) -> (-129.1273, 354.3935) centre (-129.1273, 374.4912) ccw
  line L230 (-129.1273, 354.3935) -> (-112.1728, 354.3935)
  arc A319 (-112.1728, 354.3935) -> (-112.1728, 394.589) centre (-112.1728, 374.4912) ccw
  line L231 (-112.1728, 348.0435) -> (-129.1273, 348.0435)
  arc A320 (-129.1273, 348.0435) -> (-129.1273, 307.848) centre (-129.1273, 327.9457) ccw
  line L232 (-129.1273, 307.848) -> (-112.1728, 307.848)
  arc A321 (-112.1728, 307.848) -> (-112.1728, 348.0435) centre (-112.1728, 327.9457) ccw
  line L233 (-112.1728, 301.498) -> (-129.1273, 301.498)
  arc A322 (-129.1273, 301.498) -> (-129.1273, 261.3025) centre (-129.1273, 281.4002) ccw
  line L234 (-129.1273, 261.3025) -> (-112.1728, 261.3025)
  arc A323 (-112.1728, 261.3025) -> (-112.1728, 301.498) centre (-112.1728, 281.4002) ccw
  line L235 (-112.1728, 254.9525) -> (-129.1273, 254.9525)
  arc A324 (-129.1273, 254.9525) -> (-129.1273, 214.757) centre (-129.1273, 234.8547) ccw
  line L236 (-129.1273, 214.757) -> (-112.1728, 214.757)
  arc A325 (-112.1728, 214.757) -> (-112.1728, 254.9525) centre (-112.1728, 234.8547) ccw
  line L237 (-112.1728, 208.407) -> (-129.1273, 208.407)
  arc A326 (-129.1273, 208.407) -> (-129.1273, 168.2115) centre (-129.1273, 188.3092) ccw
  line L238 (-129.1273, 168.2115) -> (-112.1728, 168.2115)
  arc A327 (-112.1728, 168.2115) -> (-112.1728, 208.407) centre (-112.1728, 188.3092) ccw
  line L239 (-112.1728, 161.8615) -> (-129.1273, 161.8615)
  arc A328 (-129.1273, 161.8615) -> (-129.1273, 121.666) centre (-129.1273, 141.7637) ccw
  line L240 (-129.1273, 121.666) -> (-112.1728, 121.666)
  arc A329 (-112.1728, 121.666) -> (-112.1728, 161.8615) centre (-112.1728, 141.7637) ccw
  line L241 (-112.1728, 115.316) -> (-129.1273, 115.316)
  arc A330 (-129.1273, 115.316) -> (-129.1273, 75.1205) centre (-129.1273, 95.2182) ccw
  line L242 (-129.1273, 75.1205) -> (-112.1728, 75.1205)
  arc A331 (-112.1728, 75.1205) -> (-112.1728, 115.316) centre (-112.1728, 95.2182) ccw
  line L243 (-112.1728, 68.7705) -> (-129.1272, 68.7705)
  arc A332 (-129.1272, 68.7705) -> (-129.1272, 28.575) centre (-129.1272, 48.6727) ccw
  line L244 (-129.1272, 28.575) -> (-112.1728, 28.575)
  arc A333 (-112.1728, 28.575) -> (-112.1728, 68.7705) centre (-112.1727, 48.6727) ccw
  line L245 (-48.6728, 487.68) -> (-65.6273, 487.68)
  arc A334 (-65.6273, 487.68) -> (-65.6273, 447.4845) centre (-65.6273, 467.5823) ccw
  line L246 (-65.6273, 447.4845) -> (-48.6728, 447.4845)
  arc A335 (-48.6728, 447.4845) -> (-48.6728, 487.68) centre (-48.6728, 467.5823) ccw
  line L247 (-48.6728, 441.1345) -> (-65.6273, 441.1345)
  arc A336 (-65.6273, 441.1345) -> (-65.6273, 400.939) centre (-65.6273, 421.0368) ccw
  line L248 (-65.6273, 400.939) -> (-48.6728, 400.939)
  arc A337 (-48.6728, 400.939) -> (-48.6728, 441.1345) centre (-48.6728, 421.0368) ccw
  line L249 (-48.6728, 394.589) -> (-65.6273, 394.589)
  arc A338 (-65.6273, 394.589) -> (-65.6273, 354.3935) centre (-65.6273, 374.4913) ccw
  line L250 (-65.6273, 354.3935) -> (-48.6728, 354.3935)
  arc A339 (-48.6728, 354.3935) -> (-48.6728, 394.589) centre (-48.6728, 374.4913) ccw
  line L251 (-48.6728, 348.0435) -> (-65.6273, 348.0435)
  arc A340 (-65.6273, 348.0435) -> (-65.6273, 307.848) centre (-65.6273, 327.9458) ccw
  line L252 (-65.6273, 307.848) -> (-48.6728, 307.848)
  arc A341 (-48.6728, 307.848) -> (-48.6728, 348.0435) centre (-48.6727, 327.9458) ccw
  line L253 (-48.6728, 301.498) -> (-65.6273, 301.498)
  arc A342 (-65.6273, 301.498) -> (-65.6273, 261.3025) centre (-65.6273, 281.4002) ccw
  line L254 (-65.6273, 261.3025) -> (-48.6728, 261.3025)
  arc A343 (-48.6728, 261.3025) -> (-48.6728, 301.498) centre (-48.6727, 281.4002) ccw
  line L255 (-48.6728, 254.9525) -> (-65.6273, 254.9525)
  arc A344 (-65.6273, 254.9525) -> (-65.6273, 214.757) centre (-65.6273, 234.8547) ccw
  line L256 (-65.6273, 214.757) -> (-48.6728, 214.757)
  arc A345 (-48.6728, 214.757) -> (-48.6728, 254.9525) centre (-48.6727, 234.8547) ccw
  line L257 (-48.6728, 208.407) -> (-65.6273, 208.407)
  arc A346 (-65.6273, 208.407) -> (-65.6273, 168.2115) centre (-65.6273, 188.3092) ccw
  line L258 (-65.6273, 168.2115) -> (-48.6728, 168.2115)
  arc A347 (-48.6728, 168.2115) -> (-48.6728, 208.407) centre (-48.6727, 188.3092) ccw
  line L259 (-48.6728, 161.8615) -> (-65.6273, 161.8615)
  arc A348 (-65.6273, 161.8615) -> (-65.6273, 121.666) centre (-65.6273, 141.7638) ccw
  line L260 (-65.6273, 121.666) -> (-48.6728, 121.666)
  arc A349 (-48.6728, 121.666) -> (-48.6728, 161.8615) centre (-48.6727, 141.7638) ccw
  line L261 (-48.6728, 115.316) -> (-65.6273, 115.316)
  arc A350 (-65.6273, 115.316) -> (-65.6273, 75.1205) centre (-65.6273, 95.2182) ccw
  line L262 (-65.6273, 75.1205) -> (-48.6728, 75.1205)
  arc A351 (-48.6728, 75.1205) -> (-48.6728, 115.316) centre (-48.6727, 95.2182) ccw
  line L263 (-48.6728, 68.7705) -> (-65.6272, 68.7705)
  arc A352 (-65.6272, 68.7705) -> (-65.6272, 28.575) centre (-65.6272, 48.6727) ccw
  line L264 (-65.6272, 28.575) -> (-48.6728, 28.575)
  arc A353 (-48.6728, 28.575) -> (-48.6728, 68.7705) centre (-48.6727, 48.6727) ccw
  point P0 (-628.65, 467.5822)
  dimension "d107" = 25.4
  dimension "d109" = 46.5455
  dimension "d110" = 63.5
  dimension "d111" = 3.175
  dimension "d114" = 46.5455
  dimension "d117" = 63.5
  constraints: 436 end point, 406 point on circle, 202 centre point, 4 horizontal, 4 parallel, 4 point on line, 4 tangent, 3 midpoint, 3 perpendicular, 1 vertical, 1006 other
  measures "d107" distance between parallel lines of L3 L11
  measures "d109" distance of L10.end L59.end
  measures "d110" distance of L59.end L60.end
  measures "d111" distance between parallel lines of L11 L65
  measures "d114" distance of A152.centre A156.centre
  measures "d117" distance of A152.centre A174.centre